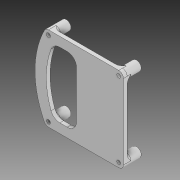
# Autodesk Inventor part: TopCase
Saved by Autodesk Inventor 2021 (Build 250183000, 183)
## iProperties
Created: 2022-08-24
Part Number: TopCase
Material: Generic
Document SubType Name: Modeling
Designer: Eli
Density: 1 g/cm^3
Appearance: Default
Author: Eli
Autodesk Inventor part; units mm, degrees
ref_plane "YZ Plane" through (0, 0, 0) normal (1, 0, 0) x (0, 1, 0)
ref_plane "XZ Plane" through (0, 0, 0) normal (0, 1, 0) x (-1, 0, 0)
ref_plane "XY Plane" through (0, 0, 0) normal (0, 0, 1) x (1, 0, 0)
sketch "Sketch1" plane through (0, 0, 0) normal (0, 0, 1) x (1, 0, 0)
  line L0 (44.1613, 40) -> (44.1613, -40) projected
  arc A0 (39.1613, -45) -> (44.1613, -40) centre (39.1613, -40) ccw projected
  line L1 (39.1613, -45) -> (-35.8387, -45) projected
  arc A1 (-39.8387, -43) -> (-35.8387, -45) centre (-35.8387, -39.9999) ccw projected
  arc A2 (-39.8387, 43) -> (-39.8387, -43) centre (44.1612, 0) ccw projected
  arc A3 (-35.8387, 45) -> (-39.8387, 43) centre (-35.8387, 40) ccw projected
  line L2 (-35.8387, 45) -> (39.1613, 45) projected
  arc A4 (44.1613, 40) -> (39.1613, 45) centre (39.1613, 40) ccw projected
  circle A5 centre (39.1613, 40) radius 2 projected
  circle A6 centre (39.1613, -40) radius 2 projected
  circle A7 centre (-35.8387, -40) radius 2 projected
  circle A8 centre (-35.8387, 40) radius 2.15 projected
  circle A9 centre (39.1613, -40) radius 5
  circle A10 centre (-35.8387, -40) radius 5
  circle A11 centre (-35.8387, 40) radius 5
  circle A12 centre (39.1613, 40) radius 5
  point P0 (0, 0)
  point P1 (-40.6387, 41.3999)
  point P2 (-39.8387, 43)
  point P3 (39.1613, 45)
  point P4 (44.1613, 40)
  point P5 (-40.6387, -41.4)
  constraints: 4 centre point, 4 coincident, 4 equal radius
extrude "Extrusion1" add sketch "Sketch1" along normal blind 15 contours A12 A4 | A0 A9 | A11 A2 A3 | A1 A2 A10
sketch "Sketch2" plane through (39.1613, -40, 15) normal (0, 0, 1) x (1, 0, 0)
  line L0 (5, 80) -> (5, 0) projected
  arc A0 (0, -5) -> (5, 0) centre (0, 0) ccw projected
  line L1 (0, -5) -> (-75, -5) projected
  arc A1 (-79, -3) -> (-75, -5) centre (-75, 0.0001) ccw projected
  arc A2 (-79, 83) -> (-79, -3) centre (5, 40) ccw projected
  arc A3 (-75, 85) -> (-79, 83) centre (-75, 80) ccw projected
  line L2 (-75, 85) -> (0, 85) projected
  arc A4 (5, 80) -> (0, 85) centre (0, 80) ccw projected
  circle A5 centre (0, 80) radius 2 projected
  circle A6 centre (0, 0) radius 2 projected
  circle A7 centre (-75, 0) radius 2 projected
  circle A8 centre (-75, 80) radius 2.15 projected
  line L3 (-69.5601, 75) -> (-45, 75)
  line L4 (-45, 75) -> (-45, 5)
  line L5 (-45, 5) -> (-69.5601, 5)
  arc A9 (-69.5601, 75) -> (-69.5601, 5) centre (5, 40) ccw
  point P0 (-39.1613, 40)
  point P1 (-79, 83)
  point P2 (-79, -3)
  dimension "d2" = 10
  dimension "d3" = 10
  dimension "d4" = 50
  dimension "d5" = 12
  constraints: 6 end point, 2 point on circle, 1 centre point, 1 horizontal, 1 parallel, 1 perpendicular
  measures "d2" distance between parallel lines of L2 L3
  measures "d3" distance between parallel lines of L1 L5
  measures "d4" distance between parallel lines of L0 L4
  measures "d5" radial gap between concentric circles of A2 A9
extrude "Extrusion2" add sketch "Sketch2" along normal blind 4
fillet "Fillet1" radius 10 4 edges at (-30.3988, -35, 17) (-5.8387, -35, 17) (-5.8387, 35, 17) (-30.3988, 35, 17)
fillet "Fillet2" radius 4 4 edges at (-32.8387, 36, 15) (-32.8387, -36, 15) (35.6257, -36.4645, 15) (35.6257, 36.4645, 15)
body "Solid1"
